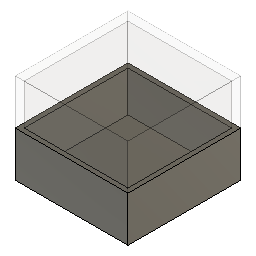
Day19Box (Autodesk Fusion 360 design; units mm, degrees)
part number: 2025-12-04-14-52-37-704
part number: 2025-12-04-18-52-37-317
part number: 2025-12-04-21-05-21-609
Autodesk Fusion 360 part; units mm, degrees
sketch "Sketch1" plane through (0, 0, 0) normal (0, 0, 1) x (1, 0, 0) in component "BoxBottom"
  line L0 (0, 0) -> (50, 0)
  line L1 (50, 0) -> (50, 50)
  line L2 (50, 50) -> (0, 50)
  line L3 (0, 50) -> (0, 0)
  dimension "d3" = 50
  dimension "d4" = 50
  constraint horizontal L0
  constraint vertical L1
  constraint horizontal L2
  constraint vertical L3
  constraint coincident L0.start L3.end
  measures "d3" distance of L0.start L2.end
  measures "d4" distance of L1.end L2.end
extrude "Extrude1" add sketch "Sketch1" along normal blind 20 makes body 1 in component "BoxBottom"
shell "Shell1" thickness 2 removed faces 1 at (16.6667, 33.3333, 20) on bodies 1 in component "BoxBottom"
sketch "Sketch1 (2)" plane through (0, 0, 0) normal (0, 0, 1) x (1, 0, 0) in component "BoxTop"
  line L0 (0, 0) -> (50, 0)
  line L1 (50, 0) -> (50, 50)
  line L2 (50, 50) -> (0, 50)
  line L3 (0, 50) -> (0, 0)
  dimension "d3_1" = 50
  dimension "d4_1" = 50
  constraint horizontal L0
  constraint vertical L1
  constraint horizontal L2
  constraint vertical L3
  constraint coincident L0.start L3.end
  measures "d3_1" distance of L0.start L2.end
  measures "d4_1" distance of L1.end L2.end
extrude "Extrude1'" add sketch "Sketch1 (2)" along normal blind 20 separate body makes body 2 in component "BoxTop"
shell "Shell1'" thickness 2 removed faces 1 at (16.6667, 33.3333, 20) on bodies 2 in component "BoxTop"
component "BoxBottom" placed x (1, 0, 0) y (0, 1, 0) z (0, 0, 1) at (0, 0, 0)
component "BoxTop" placed x (0, -1, 0) y (-1, 0, 0) z (0, 0, -1) at (50, 50, 40)
equation "Box_Width = 50 mm"
equation "Box_Height = 20 mm"
equation "d3 = Box_Width"
equation "d4 = Box_Width"
equation "d5 = Box_Height"
equation "WallThickness = 2 mm"
equation "d3_1 = Box_Width"
equation "d4_1 = Box_Width"
equation "d5_1 = Box_Height"
equation "WallThickness_1 = 2 mm"
